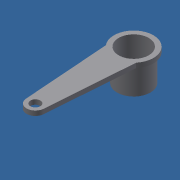
# Autodesk Inventor part: Manivelle
Saved by Autodesk Inventor 2018 (Build 220112000, 112)
## iProperties
Created: 2022-02-21
Part Number: Manivelle
Material: Generic
Document SubType Name: Modeling
Designer: Nathann
Density: 1 g/cm^3
Appearance: Default
Author: Nathann
Autodesk Inventor part; units mm, degrees
ref_plane "YZ Plane" through (0, 0, 0) normal (1, 0, 0) x (0, 1, 0)
ref_plane "XZ Plane" through (0, 0, 0) normal (0, 1, 0) x (-1, 0, 0)
ref_plane "XY Plane" through (0, 0, 0) normal (0, 0, 1) x (1, 0, 0)
sketch "Sketch1" plane through (0, 0, 0) normal (0, 0, 1) x (1, 0, 0)
  circle A0 centre (0, 0) radius 22.5
  circle A1 centre (0, 0) radius 25
  dimension "d2" = 45
  dimension "d3" = 50
  constraints: 2 centre point, 2 coincident
  measures "d2" diameter of A0
  measures "d3" diameter of A1
extrude "Extrusion1" add sketch "Sketch1" against normal blind 40
sketch "Sketch2" plane through (0, 0, 0) normal (0, 0, 1) x (1, 0, 0)
  circle A0 centre (0, 0) radius 22.5
  circle A1 centre (0, 0) radius 29.5096
  constraints: 2 centre point, 2 coincident
extrude "Extrusion2" add sketch "Sketch2" along normal blind 7
sketch "Sketch3" plane through (0, 0, 7) normal (0, 0, 1) x (1, 0, 0)
  line L0 (22.6433, -19.1315) -> (13.1623, -147.983)
  arc A0 (-13.1623, -147.983) -> (13.1623, -147.983) centre (0, -147.0145) ccw
  circle A1 centre (0, 0) radius 29.5096 projected
  line L1 (0, -29.5096) -> (0, -45.4675)
  line L2 (-22.6433, -19.1315) -> (-13.1623, -147.983)
  line L3 (-22.6433, -19.1315) -> (0, -26.0827)
  line L4 (0, -26.0827) -> (22.6433, -19.1315)
  circle A2 centre (0, -147.0145) radius 7.452
  constraints: 10 end point, 2 centre point, 2 point on circle, 2 symmetric about line, 1 coincident, 1 tangent, 1 vertical, 1 vertical alignment, 1 other
extrude "Extrusion3" add sketch "Sketch3" against normal blind 7 contours L0 A0 L2 L3 A1 L4 | A1 L3 L4 picked at (-13.395, -22.9465)
body "Solid1"
